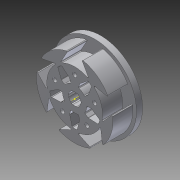
# Autodesk Inventor part: Wheel Hub
Saved by Autodesk Inventor 2013 (Build 170138000, 138)
## iProperties
Created: 2013-04-30
Part Number: Wheel Hub
Material: Task 3 Urethane
Document SubType Name: Modeling
Designer: grtstudent
Density: 1.11072 g/cm^3
Mass: 56.6592 g
Surface Area: 234.844 cm^2
Volume: 51.0112 cm^3
Author: grtstudent
Autodesk Inventor part; units mm, degrees
ref_plane "YZ Plane" through (0, 0, 0) normal (1, 0, 0) x (0, 1, 0)
ref_plane "XZ Plane" through (0, 0, 0) normal (0, 1, 0) x (-1, 0, 0)
ref_plane "XY Plane" through (0, 0, 0) normal (0, 0, 1) x (1, 0, 0)
sketch "Sketch1" plane through (0, 0, 0) normal (0, 0, 1) x (1, 0, 0)
  circle A0 centre (0, 0) radius 44.45
  line L0 (0, 0) -> (0, 52.3875) construction
  line L1 (-6.35, 34.3429) -> (-13.4938, 21.5193)
  line L2 (6.35, 34.3429) -> (13.4938, 21.5193)
  line L3 (-34.6243, 4.5733) -> (-24.6358, -6.1835)
  line L4 (-30.6998, 16.6517) -> (-16.2962, 19.4831)
  line L5 (-15.049, -31.5164) -> (-1.732, -25.3409)
  line L6 (-25.3235, -24.0515) -> (-23.5654, -9.478)
  line L7 (25.3235, -24.0515) -> (23.5654, -9.478)
  line L8 (15.049, -31.5164) -> (1.732, -25.3409)
  line L9 (30.6998, 16.6517) -> (16.2962, 19.4831)
  line L10 (34.6243, 4.5733) -> (24.6358, -6.1835)
  arc A1 (13.4938, 21.5193) -> (-13.4938, 21.5193) centre (0, 0) ccw
  arc A2 (24.6358, -6.1835) -> (16.2962, 19.4831) centre (0, 0) ccw
  arc A3 (1.732, -25.3409) -> (23.5654, -9.478) centre (0, 0) ccw
  arc A4 (-16.2962, 19.4831) -> (-24.6358, -6.1835) centre (0, 0) ccw
  arc A5 (-23.5654, -9.478) -> (-1.732, -25.3409) centre (0, 0) ccw
  arc A6 (-6.35, 34.3429) -> (-30.6998, 16.6517) centre (0, 0) ccw
  arc A7 (30.6998, 16.6517) -> (6.35, 34.3429) centre (0, 0) ccw
  arc A8 (25.3235, -24.0515) -> (34.6243, 4.5733) centre (0, 0) ccw
  arc A9 (-34.6243, 4.5733) -> (-25.3235, -24.0515) centre (0, 0) ccw
  arc A10 (-15.049, -31.5164) -> (15.049, -31.5164) centre (0, 0) ccw
  dimension "d8" = 360
  dimension "d0" = 88.9
  dimension "d4" = 12.7
  dimension "d5" = 26.9875
  dimension "d10" = 25.4
  dimension "d11" = 9.525
  constraints: 22 end point, 20 point on circle, 11 centre point, 3 coincident, 2 symmetric about line, 1 vertical, 31 other
  measures "d0" diameter of A0
  measures "d4" distance of L1.start L2.start
  measures "d5" distance of L2.end L1.end
  measures "d10" radius of A4
  measures "d11" radial gap between concentric circles of A0 A6
extrude "Extrusion1" add sketch "Sketch1" along normal blind 19.05 contours L1 A1 L2 A7 L9 A2 L10 A8 L7 A3 L8 A10 L5 A5 L6 A9 L3 A4 L4 A6
fillet "Fillet3" radius 0.5953 10 edges at (16.2962, 19.4831, 9.525) (24.6358, -6.1835, 9.525) (23.5654, -9.478, 9.525) (1.732, -25.3409, 9.525) (-1.732, -25.3409, 9.525) (-23.5654, -9.478, 9.525) (-24.6358, -6.1835, 9.525) (-16.2962, 19.4831, 9.525) (-13.4938, 21.5193, 9.525) (13.4938, 21.5193, 9.525)
fillet "Fillet3" radius 0.5953 10 edges at (-6.35, 34.3429, 9.525) (-34.6243, 4.5733, 9.525) (-25.3235, -24.0515, 9.525) (-30.6998, 16.6517, 9.525) (-15.049, -31.5164, 9.525) (6.35, 34.3429, 9.525) (30.6998, 16.6517, 9.525) (34.6243, 4.5733, 9.525) (25.3235, -24.0515, 9.525) (15.049, -31.5164, 9.525)
sketch "Sketch8" plane through (0, 0, 0) normal (0, 0, -1) x (-1, 0, 0)
  circle A0 centre (0, 0) radius 38.1
  arc A1 (-13.873, -30.9711) -> (-13.8588, -32.0576) centre (-13.6226, -31.5111) ccw projected
  arc A2 (-13.8588, -32.0576) -> (13.8588, -32.0576) centre (0, 0) ccw projected
  arc A3 (13.8588, -32.0576) -> (13.873, -30.9711) centre (13.6226, -31.5111) ccw projected
  line L0 (3.6675, -26.2384) -> (13.873, -30.9711) projected
  arc A4 (3.8282, -25.1098) -> (3.6675, -26.2384) centre (3.918, -25.6984) ccw projected
  arc A5 (3.8282, -25.1098) -> (22.6979, -11.4002) centre (0, 0) ccw projected
  arc A6 (23.8209, -11.5961) -> (22.6979, -11.4002) centre (23.2299, -11.6674) ccw projected
  line L1 (25.1682, -22.7646) -> (23.8209, -11.5961) projected
  arc A7 (25.1682, -22.7646) -> (26.206, -23.0869) centre (25.7593, -22.6933) ccw projected
  arc A8 (26.206, -23.0869) -> (34.7712, 3.2742) centre (0, 0) ccw projected
  arc A9 (34.7712, 3.2742) -> (33.7423, 3.6235) centre (34.1785, 3.2184) ccw projected
  line L2 (26.0876, -4.6201) -> (33.7423, 3.6235) projected
  arc A10 (25.0639, -4.1185) -> (26.0876, -4.6201) centre (25.6513, -4.215) ccw projected
  arc A11 (25.0639, -4.1185) -> (17.8563, 18.0641) centre (0, 0) ccw projected
  arc A12 (18.3896, 19.0716) -> (17.8563, 18.0641) centre (18.2748, 18.4875) ccw projected
  line L3 (29.4279, 16.9018) -> (18.3896, 19.0716) projected
  arc A13 (29.4279, 16.9018) -> (30.055, 17.7891) centre (29.5427, 17.4859) ccw projected
  arc A14 (30.055, 17.7891) -> (7.631, 34.0811) centre (0, 0) ccw projected
  arc A15 (7.631, 34.0811) -> (6.9808, 33.2105) centre (7.5009, 33.5002) ccw projected
  line L4 (12.4555, 23.383) -> (6.9808, 33.2105) projected
  arc A16 (11.6621, 22.5645) -> (12.4555, 23.383) centre (11.9354, 23.0933) ccw projected
  arc A17 (11.6621, 22.5645) -> (-11.6621, 22.5645) centre (0, 0) ccw projected
  arc A18 (-12.4555, 23.383) -> (-11.6621, 22.5645) centre (-11.9354, 23.0933) ccw projected
  line L5 (-6.9808, 33.2105) -> (-12.4555, 23.383) projected
  arc A19 (-6.9808, 33.2105) -> (-7.631, 34.0811) centre (-7.5009, 33.5002) ccw projected
  arc A20 (-7.631, 34.0811) -> (-30.055, 17.7891) centre (0, 0) ccw projected
  arc A21 (-30.055, 17.7891) -> (-29.4279, 16.9018) centre (-29.5427, 17.4859) ccw projected
  line L6 (-18.3896, 19.0716) -> (-29.4279, 16.9018) projected
  arc A22 (-17.8563, 18.0641) -> (-18.3896, 19.0716) centre (-18.2748, 18.4875) ccw projected
  arc A23 (-17.8563, 18.0641) -> (-25.0639, -4.1185) centre (0, 0) ccw projected
  arc A24 (-26.0876, -4.6201) -> (-25.0639, -4.1185) centre (-25.6513, -4.215) ccw projected
  line L7 (-33.7423, 3.6235) -> (-26.0876, -4.6201) projected
  arc A25 (-33.7423, 3.6235) -> (-34.7712, 3.2742) centre (-34.1785, 3.2184) ccw projected
  arc A26 (-34.7712, 3.2742) -> (-26.206, -23.0869) centre (0, 0) ccw projected
  arc A27 (-26.206, -23.0869) -> (-25.1682, -22.7646) centre (-25.7593, -22.6933) ccw projected
  line L8 (-23.8209, -11.5961) -> (-25.1682, -22.7646) projected
  arc A28 (-22.6979, -11.4002) -> (-23.8209, -11.5961) centre (-23.2299, -11.6674) ccw projected
  arc A29 (-22.6979, -11.4002) -> (-3.8282, -25.1098) centre (0, 0) ccw projected
  arc A30 (-3.6675, -26.2384) -> (-3.8282, -25.1098) centre (-3.918, -25.6984) ccw projected
  line L9 (-13.873, -30.9711) -> (-3.6675, -26.2384) projected
  dimension "d55" = 3.175
  constraints: 1 centre point, 1 coincident
  measures "d55" radial gap between concentric circles of A20 A0
extrude "Extrusion5" add sketch "Sketch8" along normal blind 3.175 contours A0 | L9 A30 A29 A28 L8 A27 A26 A25 L7 A24 A23 A22 L6 A21 A20 A19 L5 A18 A17 A16 L4 A15 A14 A13 L3 A12 A11 A10 L2 A9 A8 A7 L1 A6 A5 A4 L0 A3 A2 A1
sketch "Sketch9" plane through (0, 0, 19.05) normal (0, 0, 1) x (1, 0, 0)
  line L0 (3.2079, 5.5562) -> (6.4158, 0)
  line L1 (6.4158, 0) -> (3.2079, -5.5562)
  line L2 (3.2079, -5.5562) -> (-3.2079, -5.5562)
  line L3 (-3.2079, -5.5562) -> (-6.4158, 0)
  line L4 (-6.4158, 0) -> (-3.2079, 5.5562)
  line L5 (-3.2079, 5.5562) -> (3.2079, 5.5562)
  point P0 (0, 0)
  point P1 (0, 0)
  dimension "d58" = 11.1125
  constraints: 12 end point, 1 coincident, 1 horizontal, 13 other
  measures "d58" distance between parallel lines of L2 L5
extrude "Extrusion6" cut sketch "Sketch9" against normal blind 25.4
sketch "Sketch10" plane through (0, 0, 19.05) normal (0, 0, 1) x (1, 0, 0)
  line L0 (0, 0) -> (0, 22.225) construction
  point P0 (0, 19.05)
  point P1 (-18.1176, 5.8868)
  point P2 (-11.1973, -15.4118)
  point P3 (11.1973, -15.4118)
  point P4 (18.1176, 5.8868)
  dimension "d61" = 19.05
  dimension "d64" = 360
  constraints: 2 end point, 1 point on line, 1 vertical, 6 other
  measures "d61" distance of L0.start point (0, 19.05)
hole "Hole2" at (0, 19.05, 19.05) at (-18.1176, 5.8868, 19.05) at (-11.1973, -15.4118, 19.05) at (11.1973, -15.4118, 19.05) at (18.1176, 5.8868, 19.05) direction (0, 0, -1) diameter 3.81 depth 25.4 tip angle 118 clearance for "Socket Head Cap Screw" size "#6" standard "Ansi Unified Screw Threads"
sketch "Sketch20" plane through (0, 0, 19.05) normal (0, 0, 1) x (1, 0, 0)
  point P0 (0, 0)
sketch "Sketch21" plane through (0, 0, 0) normal (0, 0, 1) x (1, 0, 0)
  circle A0 centre (0, 0) radius 38.1 projected
  arc A1 (-26.206, -23.0869) -> (-25.1682, -22.7646) centre (-25.7593, -22.6933) ccw projected
  arc A2 (-34.7712, 3.2742) -> (-26.206, -23.0869) centre (0, 0) ccw projected
  arc A3 (-33.7423, 3.6235) -> (-34.7712, 3.2742) centre (-34.1785, 3.2184) ccw projected
  line L0 (-26.0876, -4.6201) -> (-33.7423, 3.6235) projected
  arc A4 (-26.0876, -4.6201) -> (-25.0639, -4.1185) centre (-25.6513, -4.215) ccw projected
  arc A5 (-17.8563, 18.0641) -> (-25.0639, -4.1185) centre (0, 0) ccw projected
  arc A6 (-17.8563, 18.0641) -> (-18.3896, 19.0716) centre (-18.2748, 18.4875) ccw projected
  line L1 (-29.4279, 16.9018) -> (-18.3896, 19.0716) projected
  arc A7 (-30.055, 17.7891) -> (-29.4279, 16.9018) centre (-29.5427, 17.4859) ccw projected
  arc A8 (-7.631, 34.0811) -> (-30.055, 17.7891) centre (0, 0) ccw projected
  arc A9 (-6.9808, 33.2105) -> (-7.631, 34.0811) centre (-7.5009, 33.5002) ccw projected
  line L2 (-12.4555, 23.383) -> (-6.9808, 33.2105) projected
  arc A10 (-12.4555, 23.383) -> (-11.6621, 22.5645) centre (-11.9354, 23.0933) ccw projected
  arc A11 (11.6621, 22.5645) -> (-11.6621, 22.5645) centre (0, 0) ccw projected
  arc A12 (11.6621, 22.5645) -> (12.4555, 23.383) centre (11.9354, 23.0933) ccw projected
  line L3 (6.9808, 33.2105) -> (12.4555, 23.383) projected
  arc A13 (7.631, 34.0811) -> (6.9808, 33.2105) centre (7.5009, 33.5002) ccw projected
  arc A14 (30.055, 17.7891) -> (7.631, 34.0811) centre (0, 0) ccw projected
  arc A15 (29.4279, 16.9018) -> (30.055, 17.7891) centre (29.5427, 17.4859) ccw projected
  line L4 (18.3896, 19.0716) -> (29.4279, 16.9018) projected
  arc A16 (18.3896, 19.0716) -> (17.8563, 18.0641) centre (18.2748, 18.4875) ccw projected
  arc A17 (25.0639, -4.1185) -> (17.8563, 18.0641) centre (0, 0) ccw projected
  arc A18 (25.0639, -4.1185) -> (26.0876, -4.6201) centre (25.6513, -4.215) ccw projected
  line L5 (33.7423, 3.6235) -> (26.0876, -4.6201) projected
  arc A19 (34.7712, 3.2742) -> (33.7423, 3.6235) centre (34.1785, 3.2184) ccw projected
  arc A20 (26.206, -23.0869) -> (34.7712, 3.2742) centre (0, 0) ccw projected
  arc A21 (25.1682, -22.7646) -> (26.206, -23.0869) centre (25.7593, -22.6933) ccw projected
  line L6 (23.8209, -11.5961) -> (25.1682, -22.7646) projected
  arc A22 (23.8209, -11.5961) -> (22.6979, -11.4002) centre (23.2299, -11.6674) ccw projected
  arc A23 (3.8282, -25.1098) -> (22.6979, -11.4002) centre (0, 0) ccw projected
  arc A24 (3.8282, -25.1098) -> (3.6675, -26.2384) centre (3.918, -25.6984) ccw projected
  line L7 (13.873, -30.9711) -> (3.6675, -26.2384) projected
  arc A25 (13.8588, -32.0576) -> (13.873, -30.9711) centre (13.6226, -31.5111) ccw projected
  arc A26 (-13.8588, -32.0576) -> (13.8588, -32.0576) centre (0, 0) ccw projected
  arc A27 (-13.873, -30.9711) -> (-13.8588, -32.0576) centre (-13.6226, -31.5111) ccw projected
  line L8 (-3.6675, -26.2384) -> (-13.873, -30.9711) projected
  arc A28 (-3.6675, -26.2384) -> (-3.8282, -25.1098) centre (-3.918, -25.6984) ccw projected
  arc A29 (-22.6979, -11.4002) -> (-3.8282, -25.1098) centre (0, 0) ccw projected
  arc A30 (-22.6979, -11.4002) -> (-23.8209, -11.5961) centre (-23.2299, -11.6674) ccw projected
  line L9 (-25.1682, -22.7646) -> (-23.8209, -11.5961) projected
extrude "Extrusion12" add sketch "Sketch21" along normal blind 0.7937
sketch "Sketch22" plane through (0, 0, 19.05) normal (0, 0, 1) x (1, 0, 0)
  circle A0 centre (11.1973, -15.4118) radius 1.905 projected
  circle A1 centre (-11.1973, -15.4118) radius 1.905 projected
  line L0 (8.6739, -19.2372) -> (6.6227, -15.1391)
  line L1 (6.6227, -15.1391) -> (9.1461, -11.3137)
  line L2 (9.1461, -11.3137) -> (13.7207, -11.5864)
  line L3 (13.7207, -11.5864) -> (15.7719, -15.6844)
  line L4 (15.7719, -15.6844) -> (13.2485, -19.5098)
  line L5 (13.2485, -19.5098) -> (8.6739, -19.2372)
  line L6 (-8.6739, -19.2372) -> (-13.2485, -19.5098)
  line L7 (-13.2485, -19.5098) -> (-15.7719, -15.6844)
  line L8 (-15.7719, -15.6844) -> (-13.7207, -11.5864)
  line L9 (-13.7207, -11.5864) -> (-9.1461, -11.3137)
  line L10 (-9.1461, -11.3137) -> (-6.6227, -15.1391)
  line L11 (-6.6227, -15.1391) -> (-8.6739, -19.2372)
  arc A2 (-1.6784, -23.435) -> (1.6784, -23.435) centre (0, 0) ccw
  arc A3 (-2.7815, -10.7588) -> (2.7815, -10.7588) centre (0, 0) ccw
  line L12 (4.5231, -14.3404) -> (3.7082, -11.2993)
  line L13 (-4.5231, -14.3404) -> (-3.7082, -11.2993)
  line L14 (0, 0) -> (0, -31.75) construction
  arc A4 (3.8282, -25.1098) -> (22.6979, -11.4002) centre (0, 0) ccw construction
  arc A5 (-2.7815, -10.7588) -> (-3.7082, -11.2993) centre (-2.9722, -11.4965) ccw
  arc A6 (3.7082, -11.2993) -> (2.7815, -10.7588) centre (2.9722, -11.4965) ccw
  line L15 (4.5235, -14.7334) -> (2.3604, -22.8707)
  line L16 (-2.3604, -22.8707) -> (-4.5235, -14.7334)
  arc A7 (-6.278, -13.8868) -> (4.0823, -14.6831) centre (0, 0) ccw construction
  arc A8 (4.5235, -14.7334) -> (4.5231, -14.3404) centre (3.7871, -14.5376) ccw
  arc A9 (-4.5231, -14.3404) -> (-4.5235, -14.7334) centre (-3.7871, -14.5376) ccw
  arc A10 (1.6784, -23.435) -> (2.3604, -22.8707) centre (1.6239, -22.6749) ccw
  arc A11 (-2.3604, -22.8707) -> (-1.6784, -23.435) centre (-1.6239, -22.6749) ccw
  point P0 (-6.7136, -22.5154)
  point P1 (6.7136, -22.5154)
  point P2 (-3.5061, -10.5449)
  point P3 (3.5061, -10.5449)
  point P4 (4.5757, -14.5369)
  point P5 (-4.5757, -14.5369)
  point P6 (4.5757, -14.5369)
  point P7 (2.2224, -23.3897)
  point P8 (-2.2224, -23.3897)
  point P9 (0, -31.75)
  point P10 (2.2224, -23.3897)
  point P11 (-2.2224, -23.3897)
  point P12 (-6.8401, -22.9875)
  point P13 (-3.2215, -19.6312)
  point P14 (3.5269, -18.4825)
  point P15 (5.7565, -18.9437)
  point P16 (0, 2.54)
  dimension "d165" = 7.9375
  dimension "d166" = 7.9375
  dimension "d168" = 30
  dimension "d169" = 1.905
  dimension "d170" = 11.1125
  dimension "d177" = 31.75
  dimension "d179" = 0.762
  dimension "d180" = 0.762
  dimension "d181" = 15.24
  dimension "d182" = 0.762
  dimension "d183" = 0.762
  dimension "d184" = 2.54
  constraints: 34 end point, 31 point on circle, 20 point on line, 12 tangent, 9 centre point, 8 coincident, 2 equal radius, 1 vertical, 28 other
  measures "d165" distance between parallel lines of L2 L5
  measures "d166" distance between parallel lines of L9 L6
  measures "d168" angle of L13 L12
  measures "d169" radial gap between concentric circles of A2 A4
  measures "d170" radius of A3
  measures "d177" distance of point (0, 0) point (0, -31.75)
  measures "d179" radius of A6
  measures "d180" radius of A5
  measures "d181" radius of A7
  measures "d182" radius of A8
  measures "d183" radius of A10
  measures "d184" distance of point (0, 2.54) point (0, 0)
extrude "Extrusion13" cut sketch "Sketch22" against normal blind 25.4 contours A11 L16 A9 L13 A5 A3 A6 L12 A8 L15 A10 A2
pattern_circular "Circular Pattern5" count 5 over 360 about axis through (0, 0, 0) along (0, 0, -1) of "Extrusion13"
sketch "Sketch23" plane through (0, 0, -3.175) normal (0, 0, -1) x (-1, 0, 0)
  line L0 (-9.6004, -7.0184) -> (-12.2408, -8.7332) projected
  arc A0 (-12.6145, -8.855) -> (-12.2408, -8.7332) centre (-12.6559, -8.0941) ccw projected
  line L1 (-12.6145, -8.855) -> (-21.0219, -9.3123) projected
  arc A1 (-21.7693, -8.838) -> (-21.0219, -9.3123) centre (-21.0633, -8.5514) ccw projected
  arc A2 (-22.8066, -5.6456) -> (-21.7693, -8.838) centre (0, 0) ccw projected
  arc A3 (-22.4807, -4.8226) -> (-22.8066, -5.6456) centre (-22.067, -5.4625) ccw projected
  line L2 (-22.4807, -4.8226) -> (-15.4101, -0.2508) projected
  arc A4 (-15.0363, -0.1297) -> (-15.4101, -0.2508) centre (-14.9964, -0.8907) ccw projected
  line L3 (-15.0363, -0.1297) -> (-11.8922, 0.0351) projected
  arc A5 (-11.0917, -0.6793) -> (-11.8922, 0.0351) centre (-11.8523, -0.7259) ccw projected
  arc A6 (-11.0917, -0.6793) -> (-9.3727, -5.97) centre (0, 0) ccw projected
  arc A7 (-9.6004, -7.0184) -> (-9.3727, -5.97) centre (-10.0154, -6.3793) ccw projected
  line L4 (-9.6416, 6.9617) -> (-12.0883, 8.943) projected
  arc A8 (-12.3197, 9.2607) -> (-12.0883, 8.943) centre (-11.6088, 9.5352) ccw projected
  line L5 (-12.3197, 9.2607) -> (-15.3526, 17.1154) projected
  arc A9 (-15.1326, 17.9728) -> (-15.3526, 17.1154) centre (-14.6418, 17.3899) ccw projected
  arc A10 (-12.4169, 19.9458) -> (-15.1326, 17.9728) centre (0, 0) ccw projected
  arc A11 (-11.5335, 19.8902) -> (-12.4169, 19.9458) centre (-12.0142, 19.2989) ccw projected
  line L6 (-11.5335, 19.8902) -> (-5.0005, 14.5784) projected
  arc A12 (-4.7698, 14.2603) -> (-5.0005, 14.5784) centre (-5.4812, 13.9872) ccw projected
  line L7 (-4.7698, 14.2603) -> (-3.6415, 11.321) projected
  arc A13 (-4.0736, 10.3389) -> (-3.6415, 11.321) centre (-4.3529, 11.0479) ccw projected
  arc A14 (-4.0736, 10.3389) -> (-8.5741, 7.0691) centre (0, 0) ccw projected
  arc A15 (-9.6416, 6.9617) -> (-8.5741, 7.0691) centre (-9.162, 7.5539) ccw projected
  line L8 (3.6415, 11.321) -> (4.7698, 14.2603) projected
  arc A16 (5.0005, 14.5784) -> (4.7698, 14.2603) centre (5.4812, 13.9872) ccw projected
  line L9 (5.0005, 14.5784) -> (11.5335, 19.8902) projected
  arc A17 (12.4169, 19.9458) -> (11.5335, 19.8902) centre (12.0142, 19.2989) ccw projected
  arc A18 (15.1326, 17.9728) -> (12.4169, 19.9458) centre (0, 0) ccw projected
  arc A19 (15.3526, 17.1154) -> (15.1326, 17.9728) centre (14.6418, 17.3899) ccw projected
  line L10 (15.3526, 17.1154) -> (12.3197, 9.2607) projected
  arc A20 (12.0883, 8.943) -> (12.3197, 9.2607) centre (11.6088, 9.5352) ccw projected
  line L11 (12.0883, 8.943) -> (9.6416, 6.9617) projected
  arc A21 (8.5741, 7.0691) -> (9.6416, 6.9617) centre (9.162, 7.5539) ccw projected
  arc A22 (8.5741, 7.0691) -> (4.0736, 10.3389) centre (0, 0) ccw projected
  arc A23 (3.6415, 11.321) -> (4.0736, 10.3389) centre (4.3529, 11.0479) ccw projected
  line L12 (11.8922, 0.0351) -> (15.0363, -0.1297) projected
  arc A24 (15.4101, -0.2508) -> (15.0363, -0.1297) centre (14.9964, -0.8907) ccw projected
  line L13 (15.4101, -0.2508) -> (22.4807, -4.8226) projected
  arc A25 (22.8066, -5.6456) -> (22.4807, -4.8226) centre (22.067, -5.4625) ccw projected
  arc A26 (21.7693, -8.838) -> (22.8066, -5.6456) centre (0, 0) ccw projected
  arc A27 (21.0219, -9.3123) -> (21.7693, -8.838) centre (21.0633, -8.5514) ccw projected
  line L14 (21.0219, -9.3123) -> (12.6145, -8.855) projected
  arc A28 (12.2408, -8.7332) -> (12.6145, -8.855) centre (12.6559, -8.0941) ccw projected
  line L15 (12.2408, -8.7332) -> (9.6004, -7.0184) projected
  arc A29 (9.3727, -5.97) -> (9.6004, -7.0184) centre (10.0154, -6.3793) ccw projected
  arc A30 (9.3727, -5.97) -> (11.0917, -0.6793) centre (0, 0) ccw projected
  arc A31 (11.8922, 0.0351) -> (11.0917, -0.6793) centre (11.8523, -0.7259) ccw projected
  line L16 (3.7082, -11.2993) -> (4.5231, -14.3404) projected
  arc A32 (4.5235, -14.7334) -> (4.5231, -14.3404) centre (3.7871, -14.5376) ccw projected
  line L17 (4.5235, -14.7334) -> (2.3604, -22.8707) projected
  arc A33 (1.6784, -23.435) -> (2.3604, -22.8707) centre (1.6239, -22.6749) ccw projected
  arc A34 (-1.6784, -23.435) -> (1.6784, -23.435) centre (0, 0) ccw projected
  arc A35 (-2.3604, -22.8707) -> (-1.6784, -23.435) centre (-1.6239, -22.6749) ccw projected
  line L18 (-2.3604, -22.8707) -> (-4.5235, -14.7334) projected
  arc A36 (-4.5231, -14.3404) -> (-4.5235, -14.7334) centre (-3.7871, -14.5376) ccw projected
  line L19 (-4.5231, -14.3404) -> (-3.7082, -11.2993) projected
  arc A37 (-2.7815, -10.7588) -> (-3.7082, -11.2993) centre (-2.9722, -11.4965) ccw projected
  arc A38 (-2.7815, -10.7588) -> (2.7815, -10.7588) centre (0, 0) ccw projected
  arc A39 (3.7082, -11.2993) -> (2.7815, -10.7588) centre (2.9722, -11.4965) ccw projected
  circle A40 centre (-11.1973, -15.4118) radius 1.905 projected
  circle A41 centre (18.1176, 5.8868) radius 1.905 projected
  circle A42 centre (0, 19.05) radius 1.905 projected
  circle A43 centre (11.1973, -15.4118) radius 1.905 projected
  circle A44 centre (-18.1176, 5.8868) radius 1.905 projected
  line L20 (-3.2079, 5.5562) -> (3.2079, 5.5562) projected
  line L21 (3.2079, 5.5562) -> (6.4158, 0) projected
  line L22 (6.4158, 0) -> (3.2079, -5.5562) projected
  line L23 (3.2079, -5.5562) -> (-3.2079, -5.5562) projected
  line L24 (-3.2079, -5.5562) -> (-6.4158, 0) projected
  line L25 (-6.4158, 0) -> (-3.2079, 5.5562) projected
  circle A45 centre (0, 0) radius 38.1 projected
extrude "Extrusion14" add sketch "Sketch23" along normal blind 1.5875
sketch "Sketch24" plane through (0, 0, 19.05) normal (0, 0, 1) x (1, 0, 0)
  line L0 (-3.2079, 5.5562) -> (3.2079, 5.5562) projected
  line L1 (-3.0613, 5.3022) -> (-1.6607, 5.3022)
  line L2 (1.6607, 5.3022) -> (3.0613, 5.3022)
  arc A0 (1.6607, 5.3022) -> (-1.6607, 5.3022) centre (0, 0) ccw
  line L3 (3.0613, 5.3022) -> (3.7615, 4.0894)
  line L4 (5.4223, 1.2129) -> (6.1225, 0)
  line L5 (6.1225, 0) -> (5.4223, -1.2129)
  line L6 (3.7615, -4.0894) -> (3.0613, -5.3022)
  line L7 (3.0613, -5.3022) -> (1.6607, -5.3022)
  line L8 (-1.6607, -5.3022) -> (-3.0613, -5.3022)
  line L9 (-3.0613, -5.3022) -> (-3.7615, -4.0894)
  line L10 (-5.4223, -1.2129) -> (-6.1225, 0)
  line L11 (-6.1225, 0) -> (-5.4223, 1.2129)
  line L12 (-3.7615, 4.0894) -> (-3.0613, 5.3022)
  arc A1 (-3.7615, 4.0894) -> (-5.4223, 1.2129) centre (0, 0) ccw
  arc A2 (5.4223, 1.2129) -> (3.7615, 4.0894) centre (0, 0) ccw
  arc A3 (3.7615, -4.0894) -> (5.4223, -1.2129) centre (0, 0) ccw
  arc A4 (-5.4223, -1.2129) -> (-3.7615, -4.0894) centre (0, 0) ccw
  arc A5 (-1.6607, -5.3022) -> (1.6607, -5.3022) centre (0, 0) ccw
  line L13 (-6.4158, 0) -> (-3.2079, 5.5562) projected
  line L14 (-3.2079, -5.5562) -> (-6.4158, 0) projected
  line L15 (3.2079, -5.5562) -> (-3.2079, -5.5562) projected
  line L16 (6.4158, 0) -> (3.2079, -5.5562) projected
  line L17 (3.2079, 5.5562) -> (6.4158, 0) projected
  constraints: 24 end point, 12 point on circle, 6 centre point, 2 coincident, 2 parallel, 1 tangent, 7 other
extrude "Extrusion15" add sketch "Sketch24" against normal up to surface (23.8125 mm away) contours L0 A0 L1 L12 A1 L13 | L0 L17 A2 L3 L2 A0 | A1 L11 L10 A4 L14 L13 | L17 L16 A3 L5 L4 A2 | A4 L9 L8 A5 L15 L14 | L16 L15 A5 L7 L6 A3
equation "\"d3\" = d2"
equation "\"d2\" = 9.525"
body "Solid1"
